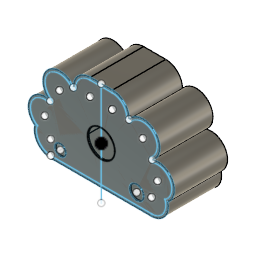
GEM_Model_f3d (Autodesk Fusion 360 design; units mm, degrees)
part number: 2026-02-15-00-40-39-643
Autodesk Fusion 360 part; units mm, degrees
sketch "Sketch1" plane through (0, 0, 0) normal (0, 1, 0) x (1, 0, 0)
  arc A0 (-86.9603, 22.741) -> (-66.7351, -14.8631) centre (-73.884, 5.5329) ccw
  arc A1 (-36.4024, -45.3508) -> (-14.4931, -67.6852) centre (-14.5441, -45.822) ccw
  arc A2 (-66.7351, -14.8631) -> (-36.4024, -45.3508) centre (-54.4848, -33.0082) ccw
  line L0 (0, -67.7) -> (0, 67.7)
  arc A3 (14.4931, -67.6852) -> (36.4024, -45.3508) centre (14.5441, -45.822) ccw
  arc A4 (36.4024, -45.3508) -> (66.7351, -14.8631) centre (54.4848, -33.0082) ccw
  arc A5 (66.7351, -14.8631) -> (86.9603, 22.741) centre (73.884, 5.5329) ccw
  line L1 (-14.4931, -67.6852) -> (14.4931, -67.6852)
  circle A6 centre (-53.6227, 34.3084) radius 7.2
  circle A7 centre (46.3773, 32.3084) radius 9.2
  circle A8 centre (0, 0) radius 17.85
  line L2 (-66.0114, 49.6899) -> (66.0037, 49.6899)
  arc A9 (-66.0037, 49.6899) -> (-86.9603, 22.741) centre (-66.0168, 28.0773) ccw
  arc A10 (86.9603, 22.741) -> (66.0037, 49.6899) centre (66.0168, 28.0773) ccw
  arc A11 (-66.0055, 46.6899) -> (-83.4323, 21.5098) centre (-66.0168, 28.0773) ccw
  arc A12 (-83.4323, 21.5098) -> (-67.7275, -12.032) centre (-73.884, 5.5329) ccw
  arc A13 (-65.0565, -17.3495) -> (-67.7275, -12.032) centre (-66.7351, -14.8631) ccw
  arc A14 (-65.0565, -17.3495) -> (-38.8802, -43.6595) centre (-54.4848, -33.0082) ccw
  arc A15 (-33.403, -45.4154) -> (-38.8802, -43.6595) centre (-36.4024, -45.3508) ccw
  arc A16 (-33.403, -45.4154) -> (-14.4967, -64.6852) centre (-14.5441, -45.822) ccw
  line L3 (-14.4967, -64.6852) -> (14.4967, -64.6852)
  arc A17 (14.4967, -64.6852) -> (33.403, -45.4154) centre (14.5441, -45.822) ccw
  arc A18 (38.8802, -43.6595) -> (33.403, -45.4154) centre (36.4024, -45.3508) ccw
  arc A19 (38.8802, -43.6595) -> (65.0565, -17.3495) centre (54.4848, -33.0082) ccw
  arc A20 (67.7275, -12.032) -> (65.0565, -17.3495) centre (66.7351, -14.8631) ccw
  arc A21 (67.7275, -12.032) -> (83.4323, 21.5098) centre (73.884, 5.5329) ccw
  arc A22 (83.4323, 21.5098) -> (66.0046, 46.6899) centre (66.0168, 28.0773) ccw
  line L4 (-66.0114, 46.6899) -> (66.0046, 46.6899)
  dimension "d19" = 14.4
  dimension "d21" = 18.4
  dimension "d24" = 35.7
  dimension "d26" = -3
  constraint symmetric A0 L0 A5
  constraint symmetric A0.end L0 A4.end
  constraint symmetric A1.start L0 A3.end
  constraint symmetric A1 L0 A3
  constraint symmetric A2 L0 A4
  constraint symmetric A1.end L0 A3.start
  constraint coincident A8.centre origin
  constraint coincident L2.start A9
  constraint coincident L2 A9.start
  constraint symmetric L0 A9.start L2.end
  constraint symmetric L0 A9 A10
  constraint symmetric L0 A0.start A5.end
  measures "d19" diameter of A6
  measures "d21" diameter of A7
  measures "d24" diameter of A8
extrude "Extrude2" add sketch "Sketch1" along normal blind 1.7 contours L0 A8 L3 A17 A18 A19 A20 A21 A22 L4 | L0 A8 A11 A12 A13 A14 A15 A16 L3 L4
extrude "Extrude3" add sketch "Sketch1" along normal blind 70 contours A0 A1 A2 L0 L1 L2 A9 A11 A12 A13 A14 A15 A16 L3 L4 | L0 A3 A4 A5 L1 L2 A10 L3 A17 A18 A19 A20 A21 A22 L4
